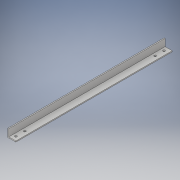
# Autodesk Inventor part: Part2
Saved by Autodesk Inventor 2017 (Build 210142000, 142)
## iProperties
Created: 2018-10-17
Part Number: Part2
Material: Generic
Document SubType Name: Modeling
Designer: ddeboer
Density: 1 g/cm^3
Appearance: Default
Author: ddeboer
Autodesk Inventor part; units mm, degrees
ref_plane "YZ Plane" through (0, 0, 0) normal (1, 0, 0) x (0, 1, 0)
ref_plane "XZ Plane" through (0, 0, 0) normal (0, 1, 0) x (-1, 0, 0)
ref_plane "XY Plane" through (0, 0, 0) normal (0, 0, 1) x (1, 0, 0)
sketch "Sketch1" plane through (0, 0, 0) normal (0, 0, 1) x (1, 0, 0)
  line L0 (0, 25.4) -> (0, 0)
  line L1 (0, 0) -> (25.4, 0)
  line L2 (3.175, 25.4) -> (3.175, 4.953)
  line L3 (4.953, 3.175) -> (25.4, 3.175)
  line L4 (0, 25.4) -> (3.175, 25.4)
  line L5 (25.4, 3.175) -> (25.4, 0)
  line L6 (3.175, 4.953) -> (3.175, 3.175)
  line L7 (4.953, 3.175) -> (3.175, 3.175)
  dimension "d0" = 25.4
  dimension "d1" = 25.4
  dimension "d2" = 3.175
  constraints: 18 end point, 3 perpendicular, 3 vertical, 2 point on line, 1 horizontal, 1 other
  measures "d0" distance of L0.start L0.end
  measures "d1" distance of L0.end L1.end
  measures "d2" distance between parallel lines of L2 L0
extrude "Extrusion1" add sketch "Sketch1" along normal blind 492.125
sketch "Sketch2" plane through (3.175, 3.175, 0) normal (0, 1, 0) x (1, 0, 0)
  circle A0 centre (9.525, -479.425) radius 2.8398
  line L0 (22.225, -492.125) -> (0, -492.125) projected
  line L1 (22.225, 0) -> (22.225, -492.125) projected
  circle A1 centre (9.525, -12.7) radius 2.8398
  line L2 (22.225, 0) -> (0, 0) projected
  point P0 (-3.175, 0)
  point P1 (1.778, -492.125)
  point P2 (1.778, 0)
  dimension "d5" = 12.7
  dimension "d6" = 12.7
  dimension "d9" = 466.725
  dimension "d31" = 12.7
  constraints: 2 centre point, 1 vertical, 2 other
  measures "d5" distance from line of A0.centre L0
  measures "d6" distance from line of A0.centre L1
  measures "d9" distance of A0.centre A1.centre
  measures "d31" distance from line of A1.centre L2
hole "Hole1" at (12.7, 3.175, 479.425) at (12.7, 3.175, 12.7) direction (0, -1, 0) diameter 6.7564 depth 25.4 tip angle 118 clearance for "Flat Head Machine Screw (82)" size "1/4" standard "Ansi Unified Screw Threads"
sketch "Sketch8" plane through (3.175, 3.175, 0) normal (0, 1, 0) x (1, 0, 0)
  circle A0 centre (9.525, -451.485) radius 5.9545
  line L0 (22.225, 0) -> (22.225, -492.125) projected
  line L1 (22.225, -492.125) -> (0, -492.125) projected
  point P0 (-3.175, 0)
  dimension "d59" = 12.7
  dimension "d60" = 40.64
  constraints: 1 centre point
  measures "d59" distance from line of A0.centre L0
  measures "d60" distance from line of A0.centre L1
hole "Hole5" at (12.7, 3.175, 451.485) direction (0, -1, 0) diameter 6.7564 depth 25.4 tip angle 118 clearance for "Flat Head Machine Screw (82)" size "1/4" standard "Ansi Unified Screw Threads"
sketch "Sketch9" plane through (3.175, 3.175, 0) normal (0, 1, 0) x (1, 0, 0)
  circle A0 centre (9.525, -40.64) radius 2.391
  line L0 (22.225, 0) -> (22.225, -492.125) projected
  line L1 (22.225, 0) -> (0, 0) projected
  point P0 (-3.175, 0)
  dimension "d68" = 12.7
  dimension "d69" = 40.64
  constraints: 1 centre point
  measures "d68" distance from line of A0.centre L0
  measures "d69" distance from line of A0.centre L1
hole "Hole6" at (12.7, 3.175, 40.64) direction (0, -1, 0) diameter 6.7564 depth 25.4 tip angle 118 clearance for "Flat Head Machine Screw (82)" size "1/4" standard "Ansi Unified Screw Threads"
body "Solid1"
